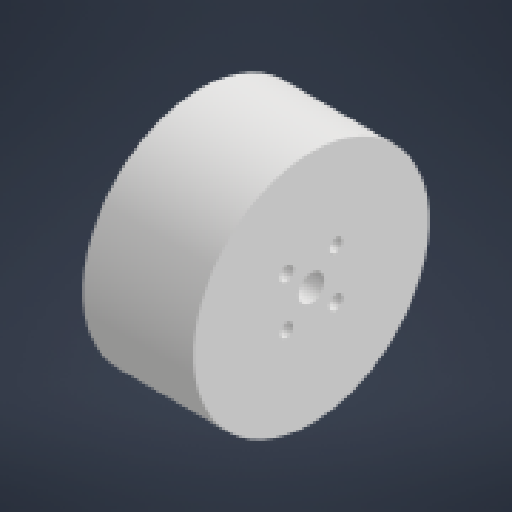
# Autodesk Inventor part: 60mm_Grip_Wheel
Saved by Autodesk Inventor 2023 (Build 270158000, 158)
## iProperties
Created: 2023-08-02
Part Number: 60mm_Grip_Wheel
Material: Generic
Document SubType Name: Modeling
Designer: izack
Density: 1 g/cm^3
Appearance: Default
Author: izack
Autodesk Inventor part; units mm, degrees
ref_plane "YZ Plane" through (0, 0, 0) normal (1, 0, 0) x (0, 1, 0)
ref_plane "XZ Plane" through (0, 0, 0) normal (0, 1, 0) x (-1, 0, 0)
ref_plane "XY Plane" through (0, 0, 0) normal (0, 0, 1) x (1, 0, 0)
sketch "Sketch1" plane through (0, 0, 0) normal (1, 0, 0) x (0, 1, 0)
  circle A0 centre (0, 0) radius 27
  circle A1 centre (0, 0) radius 8 construction
  line L0 (-8, 8) -> (8, 8) construction
  line L1 (8, 8) -> (8, -8) construction
  line L2 (8, -8) -> (-8, -8) construction
  line L3 (-8, -8) -> (-8, 8) construction
  line L4 (-8, 8) -> (8, -8) construction
  line L5 (8, 8) -> (-8, -8) construction
  circle A2 centre (5.6569, 5.6569) radius 1.6
  circle A3 centre (5.6569, -5.6569) radius 1.5
  circle A4 centre (-5.6569, -5.6569) radius 1.6
  circle A5 centre (-5.6569, 5.6569) radius 1.5
  circle A6 centre (0, 0) radius 3
  dimension "d0" = 54
  dimension "d1" = 16
  dimension "d2" = 3.2
  dimension "d3" = 3
  dimension "d4" = 3.2
  dimension "d5" = 3
  dimension "d6" = 6
  dimension "d7" = 16
  dimension "d8" = 16
  constraints: 12 end point, 7 centre point, 4 point on circle, 4 point on line, 3 coincident, 2 midpoint, 2 parallel, 1 horizontal, 1 perpendicular
  measures "d0" diameter of A0
  measures "d1" diameter of A1
  measures "d2" diameter of A2
  measures "d3" diameter of A3
  measures "d4" diameter of A4
  measures "d5" diameter of A5
  measures "d6" diameter of A6
  measures "d7" distance of L0.end L1.end
  measures "d8" distance of L1.end L2.end
extrude "Extrusion1" add sketch "Sketch1" along normal blind 25.4
body "Solid1"
